Autodesk Fusion 360 part; units mm, degrees
(part 4 of 4)
  constraint symmetric A49 L146 A161
  constraint symmetric A50 L146 A119
  constraint symmetric A51 L146 A143
  constraint symmetric A52 L146 A206
  constraint symmetric A53 L146 A214
  constraint symmetric A54 L146 A188
  constraint symmetric A55 L146 A126
  constraint symmetric A56 L146 A191
  constraint symmetric A57 L146 A129
  constraint symmetric A58 L146 A175
  constraint symmetric A59 L146 A139
  constraint symmetric A60 L146 A192
  constraint symmetric A61 L146 A170
  constraint symmetric A62 L146 A151
  constraint symmetric A63 L146 A142
  constraint symmetric A64 L146 A141
  constraint symmetric A65 L146 A204
  constraint symmetric A66 L146 A145
  constraint symmetric A67 L146 A184
  constraint symmetric A68 L146 A213
  constraint symmetric A69 L146 A200
  constraint symmetric A70 L146 A185
  constraint symmetric A71 L146 A154
  constraint symmetric A72 L146 A181
  constraint symmetric A73 L146 A165
  constraint symmetric A74 L146 A136
  constraint symmetric A75 L146 A177
  constraint symmetric A76 L146 A190
  constraint symmetric A77 L146 A202
  constraint symmetric A78 L146 A164
  constraint symmetric A79 L146 A130
  constraint symmetric A80 L146 A138
  constraint symmetric A81 L146 A205
  constraint symmetric A82 L146 A169
  constraint symmetric A83 L146 A114
  constraint symmetric A84 L146 A140
  constraint symmetric A85 L146 A108
  constraint symmetric A86 L146 A215
  constraint symmetric A87 L146 A160
  constraint symmetric A88 L146 A203
  constraint symmetric A89 L146 A179
  constraint symmetric A90 L146 A131
  constraint symmetric A91 L146 A125
  constraint symmetric A92 L146 A163
  constraint symmetric A93 L146 A124
  constraint symmetric A94 L146 A186
  constraint symmetric A95 L146 A123
  constraint symmetric A96 L146 A189
  constraint symmetric A97 L146 A173
  constraint symmetric A98 L146 A183
  constraint symmetric A99 L146 A120
  constraint symmetric A100 L146 A137
  constraint symmetric A101 L146 A194
  constraint symmetric A102 L146 A144
  constraint symmetric A103 L146 A117
  constraint symmetric A104 L146 A198
  constraint symmetric A105 L146 A195
  constraint symmetric A106 L146 A196
  constraint symmetric A107 L146 A135
  measures "d129" distance of A69.centre L9
  measures "d130" radius of A78
  measures "d131" distance of P0 L15
  measures "d132" distance of P4 L6
  measures "d133" distance of P1 L92
  measures "d134" distance of P3 L18
  measures "d135" distance of P2 L42
  measures "d136" radius of A63
  measures "d137" radius of A62
  measures "d138" radius of A43
  measures "d139" radius of A14
  measures "d140" radius of A64
  measures "d141" radius of A48
  measures "d142" radius of A75
  measures "d143" radius of A67
  measures "d144" radius of A32
  measures "d145" radius of A92
  measures "d146" radius of A91
  measures "d147" radius of A57
  measures "d148" radius of A31
  measures "d149" radius of A19
  measures "d150" radius of A17
  measures "d151" distance of L82 L89
  measures "d152" distance of L14 L59
  measures "d153" distance of L16 L36
  measures "d154" distance of L99 L105
  measures "d155" distance of L126 L144
  measures "d156" distance of L70 L72
  measures "d157" distance of L26 L98
  measures "d158" radius of A53
  measures "d159" radius of A1
  measures "d160" radius of A86
  measures "d161" vertical distance of A1.end A69.end
  measures "d162" diameter of A51
  measures "d163" diameter of A79
  measures "d164" diameter of A102
  measures "d165" diameter of A42
  measures "d166" distance of A35.centre L113.start
  measures "d167" diameter of A35
extrude "Extrude4" add sketch "v3" along normal blind 1 separate body makes body 5 at (44.7753, 0, 69.73) makes body 6 at (255.2247, 0, 69.73)
move_body "Move3" bodies 5 6 to x (1, 0, 0) y (0, 1, 0) z (0, 0, 1) at (0, 0, 250)
move_body "Move4" bodies 3 4 to x (1, 0, 0) y (0, 1, 0) z (0, 0, 1) at (-17.1012, 0, -46.9845)
equation "edgeOffset = -2 mm"
equation "d8 = edgeOffset"
equation "edgeOffsetPositive = 2 mm"
equation "d18 = edgeOffsetPositive"
equation "d21 = edgeOffsetPositive"
equation "d61 = outsideRounding"
equation "d62 = outsideRounding"
equation "d64 = outsideRounding"
equation "d65 = outsideRounding"
equation "d66 = perkeyRounding"
equation "perkeyRounding = 0.5 mm"
equation "d68 = perkeyRounding"
equation "d69 = perkeyRounding"
equation "d70 = perkeyRounding"
equation "d71 = perkeyRounding"
equation "d72 = perkeyRounding"
equation "d73 = perkeyRounding"
equation "d74 = perkeyRounding"
equation "outsideRounding = 1 mm"
equation "d136 = outsideRounding"
equation "d137 = outsideRounding"
equation "d138 = outsideRounding"
equation "d139 = outsideRounding"
equation "d140 = perkeyRounding"
equation "d141 = perkeyRounding"
equation "d142 = perkeyRounding"
equation "d143 = perkeyRounding"
equation "d144 = perkeyRounding"
equation "d145 = perkeyRounding"
equation "d146 = perkeyRounding"
equation "d147 = perkeyRounding"
equation "Switch1U = 19.05 mm"
